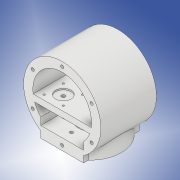
# Autodesk Inventor part: SJ003
Saved by Autodesk Inventor 2017 SP1 (Build 210196100, 196)
## iProperties
Created: 2017-06-01
Part Number: SJ003
Material: ABS Plastic
Document SubType Name: Modeling
Designer: Zach
Density: 1.06 g/cm^3
Appearance: CR White
Author: Zach
Autodesk Inventor part; units mm, degrees
ref_plane "YZ Plane" through (0, 0, 0) normal (1, 0, 0) x (0, 1, 0)
ref_plane "XZ Plane" through (0, 0, 0) normal (0, 1, 0) x (-1, 0, 0)
ref_plane "XY Plane" through (0, 0, 0) normal (0, 0, 1) x (1, 0, 0)
sketch "Sketch1" plane through (0, 0, 0) normal (0, 0, 1) x (1, 0, 0)
  circle A0 centre (0, 0) radius 62.5
  circle A1 centre (0, 0) radius 47.5
  dimension "d0" = 125
  dimension "d1" = 15
  constraints: 2 centre point, 1 coincident
  measures "d0" diameter of A0
  measures "d1" radial gap between concentric circles of A0 A1
extrude "Extrusion1" add sketch "Sketch1" along normal mid plane 90
sketch "Sketch3" plane through (0, 0, 45) normal (0, 0, 1) x (1, 0, 0)
  line L0 (34.641, -32.5) -> (34.641, -62.5)
  line L1 (34.641, -62.5) -> (-34.641, -62.5)
  line L2 (-34.641, -62.5) -> (-34.641, -32.5)
  line L3 (-34.641, -32.5) -> (34.641, -32.5)
  circle A0 centre (0, 0) radius 62.5 projected
  circle A1 centre (0, 0) radius 47.5 projected
  circle A2 centre (0, 0) radius 62.5 projected
  circle A3 centre (0, 0) radius 47.5 projected
  point P0 (0, -62.5)
  point P1 (0, -32.5)
  dimension "d87" = 30
  constraints: 8 end point, 2 midpoint, 2 perpendicular, 2 vertical alignment, 1 horizontal, 1 vertical, 5 other
  measures "d87" distance of L1.end L2.end
extrude "Extrusion3" add sketch "Sketch3" against normal blind 90 contours A1 L3 | L0 A0 L2 A1 | L0 L1 A0 | L1 L2 A0 picked at (9.1087, -34.6176) picked at (-15.536, -49.9747)
sketch "Sketch2" plane through (0, 0, 45) normal (0, 0, 1) x (1, 0, 0)
  circle A0 centre (0, 55) radius 2.5
  circle A1 centre (-47.6314, 27.5) radius 2.5
  circle A2 centre (-47.6314, -27.5) radius 2.5
  circle A3 centre (0, -55) radius 2.5
  circle A4 centre (47.6314, -27.5) radius 2.5
  circle A5 centre (47.6314, 27.5) radius 2.5
  point P0 (0, 0)
  dimension "d4" = 5
  dimension "d5" = 55
  dimension "d8" = 360
  constraints: 6 centre point, 13 other
  measures "d4" diameter of A0
  measures "d5" distance of point (0, 0) A0.centre
extrude "Extrusion2" cut sketch "Sketch2" against normal through all
sketch "Sketch17" plane through (-34.641, -62.5, 45) normal (0, -1, 0) x (1, 0, 0)
  circle A0 centre (34.641, -45) radius 50.75 construction
  line L0 (69.282, 0) -> (69.282, -90) projected
  line L1 (0, 0) -> (0, -90) projected
  line L2 (69.282, 0) -> (69.282, -90) projected
  arc A1 (69.282, -82.0886) -> (69.282, -7.9114) centre (34.641, -45) ccw
  line L3 (0, 0) -> (0, -90) projected
  arc A2 (0, -7.9114) -> (0, -82.0886) centre (34.641, -45) ccw
  line L4 (0, -7.9114) -> (0, -82.0886)
  line L5 (69.282, -7.9114) -> (69.282, -82.0886)
  dimension "d88" = 101.5
  constraints: 8 point on circle, 4 end point, 4 point on line, 3 centre point, 2 concentric, 1 coincident, 1 collinear, 1 parallel
  measures "d88" diameter of A0
extrude "Extrusion18" add sketch "Sketch17" against normal blind 27
sketch "Sketch18" plane through (-34.641, -62.5, 45) normal (0, -1, 0) x (1, 0, 0)
  circle A0 centre (34.641, -45) radius 18.5
  circle A1 centre (34.641, -45) radius 30 construction
  line L0 (34.641, -45) -> (34.641, -75) construction
  circle A2 centre (34.641, -75) radius 2.5
  circle A3 centre (60.6218, -60) radius 2.5
  circle A4 centre (60.6218, -30) radius 2.5
  circle A5 centre (34.641, -15) radius 2.5
  circle A6 centre (8.6603, -30) radius 2.5
  circle A7 centre (8.6603, -60) radius 2.5
  dimension "d92" = 60
  dimension "d91" = 37
  dimension "d93" = 5
  dimension "d96" = 360
  constraints: 7 centre point, 3 coincident, 2 end point, 1 vertical, 1 vertical alignment, 15 other
  measures "d91" diameter of A0
  measures "d93" diameter of A2
extrude "Extrusion19" cut sketch "Sketch18" against normal blind 50
sketch "Sketch19" plane through (0, 0, -45) normal (0, 0, -1) x (-1, 0, 0)
  line L0 (34.641, -32.5) -> (-34.641, -32.5) projected
  line L1 (-34.641, -32.5) -> (34.641, -32.5)
  line L2 (34.641, -32.5) -> (34.641, -44.5)
  line L3 (34.641, -44.5) -> (-34.641, -44.5)
  line L4 (-34.641, -44.5) -> (-34.641, -32.5)
  point P0 (0, 0)
  dimension "d100" = 12
  constraints: 8 end point, 2 parallel, 1 horizontal, 1 perpendicular, 1 vertical alignment
  measures "d100" distance of L1.end L2.end
extrude "Extrusion20" cut sketch "Sketch19" against normal through all
sketch "Sketch20" plane through (0, 0, -45) normal (0, 0, -1) x (-1, 0, 0)
  arc A0 (34.641, -32.5) -> (-34.641, -32.5) centre (0, 0) ccw projected
  line L0 (-47.0532, -6.5) -> (47.0532, -6.5)
  line L1 (47.0532, -6.5) -> (47.0532, -16.5)
  line L2 (47.0532, -16.5) -> (-47.0532, -16.5)
  line L3 (-47.0532, -16.5) -> (-47.0532, -6.5)
  line L4 (34.641, -44.5) -> (-34.641, -44.5) projected
  dimension "d103" = 10
  dimension "d104" = 28
  constraints: 8 end point, 2 parallel, 2 point on circle, 1 horizontal, 1 perpendicular
  measures "d103" distance of L0.end L1.end
  measures "d104" distance between parallel lines of L2 L4
extrude "Extrusion21" add sketch "Sketch20" against normal blind 90 contours L1 L2 A0 | A0 L2 L0 | A0 L2 L3
sketch "Sketch21" plane through (-47.0532, -6.5, -45) normal (0, 1, 0) x (1, 0, 0)
  line L0 (0, 0) -> (94.1063, 0) construction
  line L1 (0, -90) -> (0, 0) construction
  line L2 (94.1063, -90) -> (0, -90) construction
  line L3 (94.1063, 0) -> (94.1063, -90) construction
  circle A0 centre (47.0532, -45) radius 30.5 construction
  circle A1 centre (68.6199, -23.4332) radius 3
  line L4 (53.1199, -38.9332) -> (84.1199, -38.9332) construction
  line L5 (84.1199, -38.9332) -> (84.1199, -7.9332) construction
  line L6 (84.1199, -7.9332) -> (53.1199, -7.9332) construction
  line L7 (53.1199, -7.9332) -> (53.1199, -38.9332) construction
  line L8 (53.1199, -38.9332) -> (84.1199, -7.9332) construction
  line L9 (84.1199, -38.9332) -> (53.1199, -7.9332) construction
  line L10 (16.5532, -45) -> (77.5532, -45) construction
  line L11 (47.0532, -45) -> (68.6199, -23.4332) construction
  circle A2 centre (53.1199, -7.9332) radius 1.5
  circle A3 centre (84.1199, -7.9332) radius 1.5
  circle A4 centre (84.1199, -38.9332) radius 1.5
  circle A5 centre (53.1199, -38.9332) radius 1.5
  circle A6 centre (25.4864, -66.5668) radius 3
  line L12 (9.9864, -82.0668) -> (40.9864, -82.0668) construction
  line L13 (40.9864, -82.0668) -> (40.9864, -51.0668) construction
  line L14 (40.9864, -51.0668) -> (9.9864, -51.0668) construction
  line L15 (9.9864, -51.0668) -> (9.9864, -82.0668) construction
  line L16 (9.9864, -82.0668) -> (40.9864, -51.0668) construction
  line L17 (40.9864, -82.0668) -> (9.9864, -51.0668) construction
  circle A7 centre (9.9864, -51.0668) radius 1.5
  circle A8 centre (40.9864, -51.0668) radius 1.5
  circle A9 centre (40.9864, -82.0668) radius 1.5
  circle A10 centre (9.9864, -82.0668) radius 1.5
  line L18 (47.0532, -45) -> (25.4864, -66.5668) construction
  point P0 (94.1063, -45)
  point P1 (47.0532, -90)
  dimension "d107" = 61
  dimension "d108" = 6
  dimension "d109" = 31
  dimension "d110" = 31
  dimension "d111" = 3
  dimension "d112" = 3
  dimension "d113" = 3
  dimension "d114" = 3
  dimension "d115" = 6
  dimension "d116" = 31
  dimension "d117" = 31
  dimension "d118" = 3
  dimension "d119" = 3
  dimension "d120" = 3
  dimension "d121" = 3
  constraints: 30 end point, 11 centre point, 10 coincident, 7 midpoint, 4 parallel, 4 point on circle, 3 horizontal, 2 collinear, 2 perpendicular, 1 horizontal alignment, 1 vertical alignment
  measures "d107" diameter of A0
  measures "d108" diameter of A1
  measures "d109" distance of L6.end L5.end
  measures "d110" distance of L4.end L5.end
  measures "d111" diameter of A2
  measures "d112" diameter of A3
  measures "d113" diameter of A4
  measures "d114" diameter of A5
  measures "d115" diameter of A6
  measures "d116" distance of L15.start L14.start
  measures "d117" distance of L17.start L14.start
  measures "d118" diameter of A7
  measures "d119" diameter of A8
  measures "d120" diameter of A9
  measures "d121" diameter of A10
extrude "Extrusion22" cut sketch "Sketch21" against normal blind 15
sketch "Sketch22" plane through (-47.0532, -6.5, -45) normal (0, 1, 0) x (1, 0, 0)
  circle A0 centre (25.4864, -66.5668) radius 3 projected
  circle A1 centre (68.6199, -23.4332) radius 3 projected
  circle A2 centre (68.6199, -23.4332) radius 12.5
  circle A3 centre (25.4864, -66.5668) radius 12.5
  point P0 (47.0532, -45)
  dimension "d124" = 25
  dimension "d125" = 25
  constraints: 2 centre point, 2 coincident
  measures "d124" diameter of A2
  measures "d125" diameter of A3
extrude "Extrusion23" cut sketch "Sketch22" against normal blind 2
body "Solid1"
